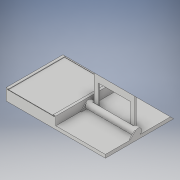
# Autodesk Inventor part: laptop
Saved by Autodesk Inventor 2019.3 (Build 233278000, 278)
## iProperties
Created: 2019-07-12
Part Number: laptop
Material: Generic
Document SubType Name: Modeling
Designer: Frienddo
Density: 1 g/cm^3
Appearance: Default
Author: Frienddo
Autodesk Inventor part; units mm, degrees
ref_plane "YZ Plane" through (0, 0, 0) normal (1, 0, 0) x (0, 1, 0)
sketch "Sketch1" plane through (0, 0, 0) normal (0, 1, 0) x (-1, 0, 0)
  line L0 (-172.25, 111.75) -> (172.25, 111.75)
  line L1 (172.25, 111.75) -> (172.25, -111.75)
  line L2 (172.25, -111.75) -> (-172.25, -111.75)
  line L3 (-172.25, -111.75) -> (-172.25, 111.75)
  line L4 (-172.25, 111.75) -> (172.25, -111.75) construction
  line L5 (172.25, 111.75) -> (-172.25, -111.75) construction
  line L6 (53.000669, 92.142184) -> (35.000669, 92.142184)
  line L7 (35.000669, 92.142184) -> (35.000669, -3.857816)
  line L8 (35.000669, -3.857816) -> (53.000669, -3.857816)
  line L9 (53.000669, -3.857816) -> (53.000669, 92.142184)
  circle A0 centre (38.000669, 83.642184) radius 1.5
  circle A1 centre (38.000669, 44.642184) radius 1.5
  circle A2 centre (38.000669, 7.642184) radius 1.5
  line L10 (146.634879, 91) -> (109.634879, 91)
  line L11 (109.634879, 91) -> (109.634879, -91)
  line L12 (109.634879, -91) -> (146.634879, -91)
  line L13 (146.634879, -91) -> (146.634879, 91)
  circle A3 centre (128.134879, 88.5) radius 1.5
  circle A4 centre (128.134879, -46.5) radius 1.5
  line L14 (89.662991, 91.78307) -> (71.662991, 91.78307)
  line L15 (71.662991, 91.78307) -> (71.662991, 57.78307)
  line L16 (71.662991, 57.78307) -> (89.662991, 57.78307)
  line L17 (89.662991, 57.78307) -> (89.662991, 91.78307)
  circle A5 centre (75.162991, 61.28307) radius 1.5
  circle A6 centre (86.162991, 86.28307) radius 1.5
  line L18 (96.694957, 29.854955) -> (71.694957, 29.854955)
  line L19 (71.694957, 29.854955) -> (71.694957, -90.145045)
  line L20 (71.694957, -90.145045) -> (96.694957, -90.145045)
  line L21 (96.694957, -90.145045) -> (96.694957, 29.854955)
  circle A7 centre (93.194957, -86.645045) radius 1.5
  circle A8 centre (93.194957, 26.354955) radius 1.5
  line L22 (-246.75, 0) -> (246.75, 0)
  line L23 (176.25, -115.75) -> (176.25, 115.75)
  line L24 (176.25, 115.75) -> (-176.25, 115.75)
  line L25 (-176.25, 115.75) -> (-176.25, -115.75)
  line L26 (-176.25, -115.75) -> (176.25, -115.75)
  line L27 (56.000669, 95.142184) -> (32.000669, 95.142184)
  line L28 (32.000669, 95.142184) -> (32.000669, -6.857816)
  line L29 (32.000669, -6.857816) -> (56.000669, -6.857816)
  line L30 (56.000669, -6.857816) -> (56.000669, 95.142184)
  line L31 (92.662991, 94.78307) -> (68.662991, 94.78307)
  line L32 (68.662991, 94.78307) -> (68.662991, 54.78307)
  line L33 (68.662991, 54.78307) -> (92.662991, 54.78307)
  line L34 (92.662991, 54.78307) -> (92.662991, 94.78307)
  line L35 (149.634879, 94) -> (106.634879, 94)
  line L36 (106.634879, 94) -> (106.634879, -94)
  line L37 (106.634879, -94) -> (149.634879, -94)
  line L38 (149.634879, -94) -> (149.634879, 94)
  line L39 (68.694957, 32.854955) -> (99.694957, 32.854955)
  line L40 (99.694957, 32.854955) -> (99.694957, -93.145045)
  line L41 (99.694957, -93.145045) -> (68.694957, -93.145045)
  line L42 (68.694957, -93.145045) -> (68.694957, 32.854955)
  line L43 (56.000669, -93.145045) -> (36.000669, -93.145045)
  line L44 (36.000669, -93.145045) -> (36.000669, -60.178685)
  line L45 (36.000669, -60.178685) -> (56.000669, -60.178685)
  line L46 (56.000669, -60.178685) -> (56.000669, -93.145045)
  point P0 (0, 0)
  dimension "d0" = 344.5
  dimension "d1" = 223.5
  dimension "d4" = 18
  dimension "d5" = 96
  dimension "d6" = 3
  dimension "d7" = 3
  dimension "d8" = 8.5
  dimension "d9" = 3
  dimension "d10" = 47.5
  dimension "d11" = 3
  dimension "d12" = 11.5
  dimension "d13" = 3
  dimension "d14" = 3
  dimension "d15" = 37
  dimension "d16" = 182
  dimension "d17" = 3
  dimension "d18" = 2.5
  dimension "d19" = 18.5
  dimension "d20" = 3
  dimension "d21" = 44.5
  dimension "d23" = 34
  dimension "d24" = 18
  dimension "d25" = 3
  dimension "d26" = 3.5
  dimension "d27" = 3.5
  dimension "d28" = 3
  dimension "d29" = 3.5
  dimension "d30" = 5.5
  dimension "d31" = 25
  dimension "d32" = 120
  dimension "d33" = 3
  dimension "d34" = 3.5
  dimension "d36" = 3
  dimension "d38" = 3.5
  dimension "d39" = 4
  dimension "d42" = 3
  dimension "d43" = 3
  dimension "d44" = 3
  dimension "d67" = 3
  dimension "d68" = 3.5
  dimension "d69" = 3.5
  dimension "d70" = 18.5
  dimension "d94" = 20
  constraints: 92 end point, 22 parallel, 11 perpendicular, 9 centre point, 6 horizontal, 2 midpoint, 16 other
  measures "d0" distance of L1.end L2.end
  measures "d1" distance of L2.end L0.start
  measures "d4" distance of L8.end L7.end
  measures "d5" distance of L6.end L7.end
  measures "d6" diameter of A0
  measures "d7" distance from line of L7 A0.centre
  measures "d8" distance from line of L6 A0.centre
  measures "d9" diameter of A1
  measures "d10" distance from line of L6 A1.centre
  measures "d11" diameter of A2
  measures "d12" distance from line of L8 A2.centre
  measures "d13" distance from line of L7 A2.centre
  measures "d14" distance from line of L7 A1.centre
  measures "d15" distance of L12.end L11.end
  measures "d16" distance of L12.end L10.start
  measures "d17" diameter of A3
  measures "d18" distance from line of L10 A3.centre
  measures "d19" distance from line of L13 A3.centre
  measures "d20" diameter of A4
  measures "d21" distance from line of L12 A4.centre
  measures "d23" distance of L16.end L14.start
  measures "d24" distance of L15.end L16.end
  measures "d25" diameter of A5
  measures "d26" distance from line of L15 A5.centre
  measures "d27" distance from line of L16 A5.centre
  measures "d28" diameter of A6
  measures "d29" distance from line of L17 A6.centre
  measures "d30" distance from line of L14 A6.centre
  measures "d31" distance of L20.end L19.end
  measures "d32" distance of L18.end L19.end
  measures "d33" diameter of A7
  measures "d34" distance from line of L20 A7.centre
  measures "d36" diameter of A8
  measures "d38" distance from line of L18 A8.centre
  measures "d39" distance between parallel lines of L1 L23
  measures "d42" distance between parallel lines of L9 L30
  measures "d43" distance between parallel lines of L17 L34
  measures "d44" distance between parallel lines of L13 L38
  measures "d67" distance between parallel lines of L18 L39
  measures "d68" distance from line of L21 A7.centre
  measures "d69" distance from line of L21 A8.centre
  measures "d70" distance from line of L13 A4.centre
  measures "d94" distance of L44.end L45.end
sketch "Sketch1 outline for Extrusion2" plane through (0, 0, 0) normal (0, 1, 0) x (-1, 0, 0)
  line L0 (-176.25, -115.75) -> (176.25, -115.75)
  line L1 (-176.25, 115.75) -> (-176.25, -115.75)
  line L2 (176.25, 115.75) -> (-176.25, 115.75)
  line L3 (176.25, -115.75) -> (176.25, 115.75)
extrude "Extrusion2" add sketch "Sketch1 outline for Extrusion2" against normal blind 2
sketch "Sketch1 outline for Extrusion3" plane through (0, 0, 0) normal (0, 1, 0) x (-1, 0, 0)
  line L0 (92.662991, 54.78307) -> (92.662991, 94.78307)
  line L1 (68.662991, 54.78307) -> (92.662991, 54.78307)
  line L2 (92.662991, 94.78307) -> (68.662991, 94.78307)
  line L3 (68.662991, 94.78307) -> (68.662991, 54.78307)
  circle A0 centre (75.162991, 61.28307) radius 1.5
  circle A1 centre (86.162991, 86.28307) radius 1.5
  line L4 (56.000669, -6.857816) -> (56.000669, 95.142184)
  line L5 (32.000669, -6.857816) -> (56.000669, -6.857816)
  line L6 (56.000669, 95.142184) -> (32.000669, 95.142184)
  line L7 (32.000669, 95.142184) -> (32.000669, -6.857816)
  circle A2 centre (38.000669, 44.642184) radius 1.5
  circle A3 centre (38.000669, 7.642184) radius 1.5
  circle A4 centre (38.000669, 83.642184) radius 1.5
  line L8 (68.694957, 32.854955) -> (99.694957, 32.854955)
  line L9 (68.694957, -93.145045) -> (68.694957, 32.854955)
  line L10 (99.694957, 32.854955) -> (99.694957, -93.145045)
  line L11 (99.694957, -93.145045) -> (68.694957, -93.145045)
  circle A5 centre (93.194957, -86.645045) radius 1.5
  line L12 (149.634879, -94) -> (149.634879, 94)
  line L13 (106.634879, -94) -> (149.634879, -94)
  line L14 (149.634879, 94) -> (106.634879, 94)
  line L15 (106.634879, 94) -> (106.634879, -94)
  circle A6 centre (128.134879, -46.5) radius 1.5
  circle A7 centre (128.134879, 88.5) radius 1.5
extrude "Extrusion3" add sketch "Sketch1 outline for Extrusion3" along normal blind 5
sketch "Sketch1 outline for Extrusion4" plane through (0, 0, 0) normal (0, 1, 0) x (-1, 0, 0)
  circle A0 centre (93.194957, -86.645045) radius 1.5
  circle A1 centre (93.194957, 26.354955) radius 1.5
extrude "Extrusion4" cut sketch "Sketch1 outline for Extrusion4" along normal blind 6
sketch "Sketch3" plane through (-32.000669, 0, -6.857816) normal (1, 0, 0) x (0, 0, -1)
  line L0 (-92, 0) -> (-92, 5) projected
  line L1 (-89, 0) -> (-89, 5) projected
  line L2 (-53, 0) -> (-53, 5) projected
  line L3 (-50, 0) -> (-50, 5) projected
  line L4 (-16, 0) -> (-16, 5) projected
  line L5 (-13, 0) -> (-13, 5) projected
  line L6 (-92, 0) -> (-89, 0)
  line L7 (-89, 0) -> (-89, 3)
  line L8 (-89, 3) -> (-92, 3)
  line L9 (-92, 3) -> (-92, 0)
  line L10 (-53, 3) -> (-50, 3)
  line L11 (-50, 3) -> (-50, 0)
  line L12 (-50, 0) -> (-53, 0)
  line L13 (-53, 0) -> (-53, 3)
  line L14 (-16, 3) -> (-13, 3)
  line L15 (-13, 3) -> (-13, 0)
  line L16 (-13, 0) -> (-16, 0)
  line L17 (-16, 0) -> (-16, 3)
  point P0 (-6.857816, 0)
  dimension "d49" = 3
  constraints: 24 end point, 6 parallel, 4 point on line, 3 horizontal, 3 perpendicular
  measures "d49" distance between parallel lines of L6 L8
sketch "Sketch3 outline for Extrusion5" plane through (-32.000669, 0, -6.857816) normal (1, 0, 0) x (0, 0, -1)
  line L0 (-92, 3) -> (-92, 0)
  line L1 (-89, 3) -> (-92, 3)
  line L2 (-89, 0) -> (-89, 3)
  line L3 (-92, 0) -> (-89, 0)
  line L4 (-53, 0) -> (-50, 0)
  line L5 (-53, 3) -> (-53, 0)
  line L6 (-50, 3) -> (-53, 3)
  line L7 (-50, 0) -> (-50, 3)
  line L8 (-16, 0) -> (-13, 0)
  line L9 (-16, 3) -> (-16, 0)
  line L10 (-13, 3) -> (-16, 3)
  line L11 (-13, 0) -> (-13, 3)
extrude "Extrusion5" cut sketch "Sketch3 outline for Extrusion5" against normal blind 6
sketch "Sketch4" plane through (-99.694957, 0, -90.145045) normal (1, 0, 0) x (0, 0, -1)
  line L0 (-115, 0) -> (-115, 5) projected
  line L1 (-118, 0) -> (-118, 5) projected
  line L2 (-5, 0) -> (-5, 5) projected
  line L3 (-5, 5) -> (-2, 5) projected
  line L4 (-2, 0) -> (-2, 5) projected
  line L5 (-118, 0) -> (-115, 0)
  line L6 (-115, 0) -> (-115, 3)
  line L7 (-115, 3) -> (-118, 3)
  line L8 (-118, 3) -> (-118, 0)
  line L9 (-5, 0) -> (-2, 0)
  line L10 (-2, 0) -> (-2, 3)
  line L11 (-2, 3) -> (-5, 3)
  line L12 (-5, 3) -> (-5, 0)
  point P0 (-90.145045, 0)
  dimension "d52" = 3
  constraints: 16 end point, 4 parallel, 2 horizontal, 2 perpendicular, 2 point on line
  measures "d52" distance between parallel lines of L5 L7
sketch "Sketch4 outline for Extrusion6" plane through (-99.694957, 0, -90.145045) normal (1, 0, 0) x (0, 0, -1)
  line L0 (-118, 3) -> (-118, 0)
  line L1 (-115, 3) -> (-118, 3)
  line L2 (-115, 0) -> (-115, 3)
  line L3 (-118, 0) -> (-115, 0)
  line L4 (-5, 3) -> (-5, 0)
  line L5 (-2, 3) -> (-5, 3)
  line L6 (-2, 0) -> (-2, 3)
  line L7 (-5, 0) -> (-2, 0)
extrude "Extrusion6" cut sketch "Sketch4 outline for Extrusion6" along normal blind 6.5
sketch "Sketch5" plane through (-68.662991, 0, 54.78307) normal (1, 0, 0) x (0, 0, -1)
  line L0 (-5, 0) -> (-5, 5) projected
  line L1 (-8, 0) -> (-8, 5) projected
  line L2 (-8, 0) -> (-5, 0)
  line L3 (-5, 0) -> (-5, 3)
  line L4 (-5, 3) -> (-8, 3)
  line L5 (-8, 3) -> (-8, 0)
  point P0 (54.78307, 0)
  dimension "d55" = 3
  constraints: 8 end point, 2 parallel, 1 horizontal, 1 perpendicular, 1 point on line
  measures "d55" distance between parallel lines of L2 L4
sketch "Sketch5 outline for Extrusion7" plane through (-68.662991, 0, 54.78307) normal (1, 0, 0) x (0, 0, -1)
  line L0 (-8, 3) -> (-8, 0)
  line L1 (-5, 3) -> (-8, 3)
  line L2 (-5, 0) -> (-5, 3)
  line L3 (-8, 0) -> (-5, 0)
extrude "Extrusion7" cut sketch "Sketch5 outline for Extrusion7" against normal blind 6.5
sketch "Sketch6" plane through (-92.662991, 0, 94.78307) normal (-1, 0, 0) x (0, 0, 1)
  line L0 (-7, 0) -> (-7, 5) projected
  line L1 (-10, 0) -> (-10, 5) projected
  line L2 (-7, 0) -> (-10, 0)
  line L3 (-10, 0) -> (-10, 3)
  line L4 (-10, 3) -> (-7, 3)
  line L5 (-7, 3) -> (-7, 0)
  point P0 (-94.78307, 0)
  dimension "d58" = 3
  constraints: 8 end point, 2 parallel, 1 horizontal, 1 perpendicular, 1 point on line
  measures "d58" distance of L4.end L0.start
sketch "Sketch6 outline for Extrusion8" plane through (-92.662991, 0, 94.78307) normal (-1, 0, 0) x (0, 0, 1)
  line L0 (-7, 0) -> (-10, 0)
  line L1 (-10, 0) -> (-10, 3)
  line L2 (-10, 3) -> (-7, 3)
  line L3 (-7, 3) -> (-7, 0)
extrude "Extrusion8" cut sketch "Sketch6 outline for Extrusion8" against normal blind 6.5
sketch "Sketch7" plane through (-149.634879, 0, 94) normal (0, 0, 1) x (1, 0, 0)
  line L0 (20, 0) -> (20, 5) projected
  line L1 (23, 0) -> (23, 5) projected
  line L2 (20, 3) -> (23, 3)
  line L3 (23, 3) -> (23, 0)
  line L4 (23, 0) -> (20, 0)
  line L5 (20, 0) -> (20, 3)
  point P0 (149.634879, 0)
  dimension "d61" = 3
  constraints: 8 end point, 2 parallel, 1 horizontal, 1 perpendicular, 1 point on line
  measures "d61" distance between parallel lines of L4 L2
sketch "Sketch7 outline for Extrusion9" plane through (-149.634879, 0, 94) normal (0, 0, 1) x (1, 0, 0)
  line L0 (20, 0) -> (23, 0)
  line L1 (20, 3) -> (20, 0)
  line L2 (23, 3) -> (20, 3)
  line L3 (23, 0) -> (23, 3)
extrude "Extrusion9" cut sketch "Sketch7 outline for Extrusion9" against normal blind 5.5
sketch "Sketch8" plane through (-106.634879, 0, -94) normal (1, 0, 0) x (0, 0, -1)
  line L0 (-49, 0) -> (-49, 5) projected
  line L1 (-46, 0) -> (-46, 5) projected
  line L2 (-49, 0) -> (-46, 0)
  line L3 (-46, 0) -> (-46, 3)
  line L4 (-46, 3) -> (-49, 3)
  line L5 (-49, 3) -> (-49, 0)
  point P0 (-94, 0)
  dimension "d64" = 3
  constraints: 8 end point, 2 parallel, 1 horizontal, 1 perpendicular, 1 point on line
  measures "d64" distance between parallel lines of L2 L4
sketch "Sketch8 outline for Extrusion10" plane through (-106.634879, 0, -94) normal (1, 0, 0) x (0, 0, -1)
  line L0 (-49, 3) -> (-49, 0)
  line L1 (-46, 3) -> (-49, 3)
  line L2 (-46, 0) -> (-46, 3)
  line L3 (-49, 0) -> (-46, 0)
extrude "Extrusion10" cut sketch "Sketch8 outline for Extrusion10" against normal up to next
sketch "Sketch9" plane through (-176.25, 0, -115.75) normal (-1, 0, 0) x (0, 0, 1)
  line L0 (231.5, 0) -> (231.5, -2) projected
  line L1 (231.5, 0) -> (231.5, 30)
  line L2 (0, 0) -> (231.5, 0) projected
  line L3 (0, 0) -> (30, 30)
  line L4 (30, 30) -> (231.5, 30)
  line L5 (0, 0) -> (231.5, 0)
  line L6 (21.75, 5) -> (209.75, 5) projected
  line L7 (189.25, 20) -> (200.25, 20)
  line L8 (200.25, 20) -> (200.25, 3)
  line L9 (200.25, 3) -> (189.25, 3)
  line L10 (189.25, 3) -> (189.25, 20)
  line L11 (189.25, 20) -> (200.25, 3) construction
  line L12 (200.25, 20) -> (189.25, 3) construction
  line L13 (137.75, 17) -> (157.75, 17)
  line L14 (157.75, 17) -> (157.75, 3)
  line L15 (157.75, 3) -> (137.75, 3)
  line L16 (137.75, 3) -> (137.75, 17)
  line L17 (137.75, 17) -> (157.75, 3) construction
  line L18 (157.75, 17) -> (137.75, 3) construction
  point P0 (115.75, 0)
  point P1 (194.75, 11.5)
  point P2 (147.75, 10)
  dimension "d71" = 30
  dimension "d72" = 45
  dimension "d100" = 15
  dimension "d101" = 62
  dimension "d102" = 17
  dimension "d103" = 14
  dimension "d104" = 20
  dimension "d105" = 2
  dimension "d106" = 2
  dimension "d107" = 11
  constraints: 32 end point, 4 horizontal, 4 midpoint, 4 parallel, 2 perpendicular, 1 vertical
  measures "d71" distance of L0.start L1.end
  measures "d72" angle of L2 L3
  measures "d100" horizontal distance of L6.end point (194.75, 11.5)
  measures "d101" horizontal distance of L6.end point (147.75, 10)
  measures "d102" distance of L7.end L8.end
  measures "d103" distance of L13.end L14.end
  measures "d104" distance of L13.start L13.end
  measures "d105" distance between parallel lines of L15 L6
  measures "d106" distance between parallel lines of L9 L6
  measures "d107" distance of L7.start L7.end
sketch "Sketch9 outline for Extrusion11" plane through (-176.25, 0, -115.75) normal (-1, 0, 0) x (0, 0, 1)
  line L0 (0, 0) -> (231.5, 0)
  line L1 (30, 30) -> (0, 0)
  line L2 (231.5, 30) -> (30, 30)
  line L3 (231.5, 0) -> (231.5, 30)
extrude "Extrusion11" add sketch "Sketch9 outline for Extrusion11" against normal blind 4
sketch "Sketch9 outline for Extrusion12" plane through (-176.25, 0, -115.75) normal (-1, 0, 0) x (0, 0, 1)
  line L0 (0, 0) -> (231.5, 0)
  line L1 (30, 30) -> (0, 0)
  line L2 (231.5, 30) -> (30, 30)
  line L3 (231.5, 0) -> (231.5, 30)
extrude "Extrusion12" add sketch "Sketch9 outline for Extrusion12" along normal blind 4 from surface at -176.25
sketch "Sketch10" plane through (0, 0, -115.75) normal (0, 0.7071068, -0.7071068) x (-1, 0, 0)
  line L0 (0, 0) -> (0, 163.69522)
  line L1 (176.25, 42.426407) -> (176.25, 0)
  line L2 (0, 0) -> (176.25, 0)
  line L3 (176.25, 0) -> (176.25, 42.426407)
  line L4 (176.25, 42.426407) -> (0, 42.426407)
  line L5 (0, 42.426407) -> (0, 0)
  point P0 (0, 81.84761)
  constraints: 8 end point, 2 parallel, 1 horizontal, 1 perpendicular
sketch "Sketch10 outline for Extrusion13" plane through (0, 0, -115.75) normal (0, 0.7071068, -0.7071068) x (-1, 0, 0)
  line L0 (0, 42.426407) -> (0, 0)
  line L1 (176.25, 42.426407) -> (0, 42.426407)
  line L2 (176.25, 0) -> (176.25, 42.426407)
  line L3 (0, 0) -> (176.25, 0)
extrude "Extrusion13" add sketch "Sketch10 outline for Extrusion13" against normal blind 4
sketch "Sketch11" plane through (-176.25, -2, 115.75) normal (0, 0, 1) x (1, 0, 0)
  line L0 (172.25, 32) -> (167.25, 32)
  line L1 (167.25, 32) -> (167.25, 30)
  line L2 (167.25, 30) -> (171.25, 30)
  line L3 (171.25, 30) -> (171.25, 27.5)
  line L4 (171.25, 27.5) -> (167.25, 27.5)
  line L5 (167.25, 27.5) -> (167.25, 25.5)
  line L6 (167.25, 25.5) -> (172.25, 25.5)
  line L7 (172.25, 2) -> (172.25, 32)
  line L8 (176.25, 32) -> (172.25, 32)
  line L9 (172.25, 32) -> (172.25, 25.5)
  line L10 (4, 32) -> (4, 2)
  line L11 (172.25, 17) -> (4, 17) construction
  line L12 (88.125, 17) -> (88.125, 10.810399) construction
  line L13 (4, 32) -> (9, 32)
  line L14 (9, 32) -> (9, 30)
  line L15 (9, 30) -> (5, 30)
  line L16 (5, 30) -> (5, 27.5)
  line L17 (5, 27.5) -> (9, 27.5)
  line L18 (9, 27.5) -> (9, 25.5)
  line L19 (9, 25.5) -> (4, 25.5)
  line L20 (4, 2) -> (4, 32)
  line L21 (0, 32) -> (4, 32)
  line L22 (4, 32) -> (4, 25.5)
  line L23 (4, 17) -> (172.25, 17) construction
  point P0 (176.25, 2)
  dimension "d79" = 2
  dimension "d80" = 2
  dimension "d81" = 2.5
  dimension "d82" = 4
  dimension "d83" = 1
  constraints: 42 end point, 10 symmetric about line, 6 perpendicular, 6 point on line, 3 midpoint, 1 horizontal, 1 vertical
  measures "d79" distance between parallel lines of L0 L2
  measures "d80" distance between parallel lines of L4 L6
  measures "d81" distance between parallel lines of L2 L4
  measures "d82" distance between parallel lines of L5 L3
  measures "d83" distance between parallel lines of L7 L3
sketch "Sketch11 outline for Extrusion14" plane through (-176.25, -2, 115.75) normal (0, 0, 1) x (1, 0, 0)
  line L0 (172.25, 25.5) -> (172.25, 32)
  line L1 (167.25, 25.5) -> (172.25, 25.5)
  line L2 (167.25, 27.5) -> (167.25, 25.5)
  line L3 (171.25, 27.5) -> (167.25, 27.5)
  line L4 (171.25, 30) -> (171.25, 27.5)
  line L5 (167.25, 30) -> (171.25, 30)
  line L6 (167.25, 32) -> (167.25, 30)
  line L7 (172.25, 32) -> (167.25, 32)
  line L8 (4, 32) -> (9, 32)
  line L9 (9, 32) -> (9, 30)
  line L10 (9, 30) -> (5, 30)
  line L11 (5, 30) -> (5, 27.5)
  line L12 (5, 27.5) -> (9, 27.5)
  line L13 (9, 27.5) -> (9, 25.5)
  line L14 (9, 25.5) -> (4, 25.5)
  line L15 (4, 25.5) -> (4, 32)
extrude "Extrusion14" add sketch "Sketch11 outline for Extrusion14" against normal up to next
sketch "Sketch12" plane through (-176.25, -2, 115.75) normal (0, 0, 1) x (1, 0, 0)
  line L0 (172.25, 27.5) -> (4, 27.5)
  line L1 (4, 27.5) -> (4, 2)
  line L2 (4, 2) -> (172.25, 2)
  line L3 (172.25, 2) -> (172.25, 27.5)
  line L4 (172.25, 2) -> (172.25, 25.5) projected
  constraints: 8 end point, 2 parallel, 1 collinear, 1 horizontal, 1 perpendicular
sketch "Sketch12 outline for Extrusion15" plane through (-176.25, -2, 115.75) normal (0, 0, 1) x (1, 0, 0)
  line L0 (4, 2) -> (4, 27.5)
  line L1 (4, 27.5) -> (172.25, 27.5)
  line L2 (172.25, 27.5) -> (172.25, 2)
  line L3 (172.25, 2) -> (4, 2)
extrude "Extrusion15" add sketch "Sketch12 outline for Extrusion15" against normal blind 4
sketch "Sketch13" plane through (-5, 25.5, -84.593146) normal (-1, 0, 0) x (0, 0, 1)
  line L0 (200.343146, 2.5) -> (0.843146, 2.5)
  line L1 (200.343146, 2.5) -> (200.343146, 0)
  line L2 (0.843146, 2.5) -> (200.343146, 2.5)
  line L3 (200.343146, 2.5) -> (200.343146, 0)
  line L4 (200.343146, 0) -> (0.843146, 0)
  line L5 (0.843146, 0) -> (0.843146, 2.5)
  point P0 (84.593146, -25.5)
  constraints: 8 end point, 2 parallel, 1 horizontal, 1 perpendicular
sketch "Sketch13 outline for Extrusion16" plane through (-5, 25.5, -84.593146) normal (-1, 0, 0) x (0, 0, 1)
  line L0 (200.343146, 2.5) -> (0.843146, 2.5)
  line L1 (200.343146, 0) -> (200.343146, 2.5)
  line L2 (0.843146, 0) -> (200.343146, 0)
  line L3 (0.843146, 2.5) -> (0.843146, 0)
extrude "Extrusion16" cut sketch "Sketch13 outline for Extrusion16" along normal up to surface (166.25 mm away)
sketch "Sketch14" plane through (-176.25, -2, 115.75) normal (-1, 0, 0) x (0, 0, 1)
  line L0 (-229.5, 0) -> (-228.671573, -0.828427)
  line L1 (-227.843146, 0) -> (-229.5, 0)
  line L2 (-229.5, 0) -> (-227.843146, 0)
  line L3 (-228.671573, -0.828427) -> (-227.843146, 0)
  line L4 (-227.843146, 0) -> (-228.671573, -0.828427)
  line L5 (-228.671573, -0.828427) -> (-229.5, 0)
  point P0 (-115.75, 2)
  constraints: 6 end point, 1 collinear, 1 horizontal, 1 perpendicular
sketch "Sketch14 outline for Extrusion17" plane through (-176.25, -2, 115.75) normal (-1, 0, 0) x (0, 0, 1)
  line L0 (-227.843146, 0) -> (-229.5, 0)
  line L1 (-228.671573, -0.828427) -> (-227.843146, 0)
  line L2 (-229.5, 0) -> (-228.671573, -0.828427)
extrude "Extrusion17" cut sketch "Sketch14 outline for Extrusion17" against normal through all
sketch "Sketch1 outline for Extrusion18" plane through (0, 0, 0) normal (0, 1, 0) x (-1, 0, 0)
  line L0 (-176.25, -115.75) -> (176.25, -115.75)
  line L1 (-176.25, 115.75) -> (-176.25, -115.75)
  line L2 (176.25, -115.75) -> (176.25, 115.75)
  line L3 (176.25, 115.75) -> (-176.25, 115.75)
  line L4 (-172.25, -111.75) -> (-172.25, 111.75)
  line L5 (172.25, -111.75) -> (-172.25, -111.75)
  line L6 (172.25, 111.75) -> (172.25, -111.75)
  line L7 (-172.25, 111.75) -> (172.25, 111.75)
extrude "Extrusion18" add sketch "Sketch1 outline for Extrusion18" against normal blind 8.6
sketch "Sketch1 outline for Extrusion19" plane through (0, 0, 0) normal (0, 1, 0) x (-1, 0, 0)
  line L0 (56.000669, -93.145045) -> (36.000669, -93.145045)
  line L1 (36.000669, -93.145045) -> (36.000669, -60.178685)
  line L2 (36.000669, -60.178685) -> (56.000669, -60.178685)
  line L3 (56.000669, -60.178685) -> (56.000669, -93.145045)
extrude "Extrusion19" cut sketch "Sketch1 outline for Extrusion19" against normal through all
sketch "Sketch15" plane through (0, -8.6, 0) normal (0, -1, 0) x (1, 0, 0)
  line L0 (-176.25, 115.75) -> (-167.25, 115.75) projected
  line L1 (176.25, 115.75) -> (176.25, -115.75) projected
  line L2 (-176.25, 115.75) -> (176.25, 115.75)
  line L3 (176.25, 115.75) -> (176.25, -115.75)
  line L4 (176.25, -115.75) -> (-176.25, -115.75)
  line L5 (-176.25, -115.75) -> (-176.25, 115.75)
  line L6 (169.25, 108.75) -> (-169.25, 108.75)
  line L7 (-169.25, 108.75) -> (-169.25, -108.75)
  line L8 (-169.25, -108.75) -> (169.25, -108.75)
  line L9 (169.25, -108.75) -> (169.25, 108.75)
  point P0 (0, 0)
  dimension "d97" = 7
  constraints: 16 end point, 4 parallel, 2 perpendicular, 1 horizontal, 3 other
  measures "d97" distance between parallel lines of L2 L6
sketch "Sketch15 outline for Extrusion20" plane through (0, -8.6, 0) normal (0, -1, 0) x (1, 0, 0)
  line L0 (-176.25, 115.75) -> (176.25, 115.75)
  line L1 (-176.25, -115.75) -> (-176.25, 115.75)
  line L2 (176.25, 115.75) -> (176.25, -115.75)
  line L3 (176.25, -115.75) -> (-176.25, -115.75)
  line L4 (169.25, -108.75) -> (169.25, 108.75)
  line L5 (169.25, 108.75) -> (-169.25, 108.75)
  line L6 (-169.25, 108.75) -> (-169.25, -108.75)
  line L7 (-169.25, -108.75) -> (169.25, -108.75)
extrude "Extrusion20" add sketch "Sketch15 outline for Extrusion20" along normal blind 3
sketch "Sketch9 outline for Extrusion21" plane through (-176.25, 0, -115.75) normal (-1, 0, 0) x (0, 0, 1)
  line L0 (189.25, 20) -> (200.25, 20)
  line L1 (200.25, 20) -> (200.25, 3)
  line L2 (200.25, 3) -> (189.25, 3)
  line L3 (189.25, 3) -> (189.25, 20)
  line L4 (137.75, 17) -> (157.75, 17)
  line L5 (157.75, 17) -> (157.75, 3)
  line L6 (157.75, 3) -> (137.75, 3)
  line L7 (137.75, 3) -> (137.75, 17)
extrude "Extrusion21" cut sketch "Sketch9 outline for Extrusion21" against normal up to surface (4 mm away)
sketch "Sketch17" plane through (176.25, 0, 115.75) normal (1, 0, 0) x (0, 0, -1)
  line L0 (231.5, 0) -> (231.5, -11.6) projected
  line L1 (231.5, -11.6) -> (231.5, 0)
  line L2 (231.5, 0) -> (243.1, -11.6)
  line L3 (243.1, -11.6) -> (231.5, -11.6)
  point P0 (115.75, 0)
  dimension "d111" = 45
  constraints: 6 end point, 1 collinear, 1 perpendicular
  measures "d111" angle of L3 L2
sketch "Sketch17 outline for Extrusion22" plane through (176.25, 0, 115.75) normal (1, 0, 0) x (0, 0, -1)
  line L0 (243.1, -11.6) -> (231.5, 0)
  line L1 (231.5, -11.6) -> (243.1, -11.6)
  line L2 (231.5, 0) -> (231.5, -11.6)
extrude "Extrusion22" add sketch "Sketch17 outline for Extrusion22" against normal up to surface (352.5 mm away)
sketch "Sketch16" plane through (176.25, 0, 115.75) normal (1, 0, 0) x (0, 0, -1)
  arc A0 (115.75, 0) -> (115.75, 20) centre (115.75, 10) ccw
  line L0 (0, 0) -> (231.5, 0)
  arc A1 (107.443376, 0) -> (115.75, 23) centre (115.75, 10) ccw
  line L1 (87.365224, 0) -> (106.557612, 19.192388)
  line L2 (115.75, 0) -> (115.75, 35.556642) construction
  arc A2 (106.557612, 19.192388) -> (107.443376, 0) centre (115.75, 10) ccw
  line L3 (87.365224, 0) -> (107.443376, 0)
  line L4 (227.5, -2) -> (4, -2)
  arc A3 (115.75, 20) -> (115.75, 0) centre (115.75, 10) ccw
  arc A4 (115.75, 23) -> (106.557612, 19.192388) centre (115.75, 10) ccw
  line L5 (115.25, 19.987492) -> (115.25, 22.990381)
  point P0 (124.942388, 19.192388)
  point P1 (139.134776, 0)
  dimension "d110" = 20
  dimension "d114" = 3
  dimension "d115" = 45
  dimension "d131" = 0.5
  constraints: 14 point on circle, 8 end point, 6 point on line, 5 centre point, 3 tangent, 2 vertical, 1 midpoint, 1 parallel
  measures "d110" diameter of A0
  measures "d114" radial gap between concentric circles of A0 A1
  measures "d115" angle of L2 L1
  measures "d131" distance between parallel lines of L2 L5
sketch "Sketch16 outline for Extrusion25" plane through (176.25, 0, 115.75) normal (1, 0, 0) x (0, 0, -1)
  line L0 (87.365224, 0) -> (106.557612, 19.192388)
  arc A0 (106.557612, 19.192388) -> (115.75, 23) centre (115.75, 10) cw
  arc A1 (115.75, 23) -> (107.443376, 0) centre (115.75, 10) cw
  line L1 (107.443376, 0) -> (87.365224, 0)
extrude "Extrusion25" add sketch "Sketch16 outline for Extrusion25" against normal blind 3
sketch "Sketch16 outline for Extrusion26" plane through (176.25, 0, 115.75) normal (1, 0, 0) x (0, 0, -1)
  circle A0 centre (115.75, 10) radius 13
  circle A1 centre (115.75, 10) radius 10
extrude "Extrusion26" add sketch "Sketch16 outline for Extrusion26" against normal blind 15
ref_plane "Work Plane1" through (88.125, 0, 115.75) normal (1, 0, 0) x (0, 0, -1)
mirror "Mirror1" about plane through (88.125, 0, 115.75) normal (1, 0, 0) of "Extrusion26", "Extrusion25"
sketch "Sketch16 outline for Extrusion27" plane through (176.25, 0, 115.75) normal (1, 0, 0) x (0, 0, -1)
  line L0 (107.443376, 0) -> (115.75, 0)
  arc A0 (106.557612, 19.192388) -> (107.443376, 0) centre (115.75, 10) ccw
  arc A1 (115.25, 22.990381) -> (106.557612, 19.192388) centre (115.75, 10) ccw
  line L1 (115.25, 19.987492) -> (115.25, 22.990381)
  arc A2 (115.75, 0) -> (115.25, 19.987492) centre (115.75, 10) cw
extrude "Extrusion27" add sketch "Sketch16 outline for Extrusion27" against normal up to surface (161.25 mm away)
ref_plane "Work Plane2" through (15.5, 0, 0) normal (1, 0, 0) x (0, 0, -1)
sketch "Sketch20" plane through (15.5, 0, 0) normal (1, 0, 0) x (0, 0, -1)
  arc A0 (0, 20) -> (0, 0) centre (0, 10) ccw
  arc A1 (0, 0) -> (0, 20) centre (0, 10) ccw
  line L0 (-115.75, 0) -> (115.75, 0)
  line L1 (127.35, -11.6) -> (115.75, 0)
  line L2 (115.75, 0) -> (1.669643, 114.080357)
  circle A2 centre (0, 10) radius 9.6
  line L3 (5.024587, 18.180069) -> (5.024587, 110.725413)
  line L4 (9.6, 10) -> (9.6, 106.15)
  dimension "d132" = 0.4
  dimension "d133" = 45
  constraints: 6 end point, 2 point on circle, 2 point on line, 1 centre point, 1 coincident, 1 collinear, 1 parallel
  measures "d132" radial gap between concentric circles of A2 A1
  measures "d133" angle of L3 L2
sketch "Sketch20 outline for Extrusion29" plane through (15.5, 0, 0) normal (1, 0, 0) x (0, 0, -1)
  line L0 (9.6, 106.15) -> (9.6, 10)
  arc A0 (9.6, 10) -> (5.024587, 18.180069) centre (0, 10) cw
  line L1 (5.024587, 18.180069) -> (5.024587, 110.725413)
  line L2 (5.024587, 110.725413) -> (9.6, 106.15)
extrude "Extrusion29" add sketch "Sketch20 outline for Extrusion29" along normal blind 15
sketch "Sketch20 outline for Extrusion30" plane through (15.5, 0, 0) normal (1, 0, 0) x (0, 0, -1)
  arc A0 (9.6, 10) -> (5.024587, 18.180069) centre (0, 10) cw
  arc A1 (5.024587, 18.180069) -> (9.6, 10) centre (0, 10) cw
extrude "Extrusion30" add sketch "Sketch20 outline for Extrusion30" against normal blind 12
sketch "Sketch21" plane through (30.5, 0, 0) normal (1, 0, 0) x (0, 0, -1)
  line L0 (5.024587, 110.725413) -> (5.024587, 18.180069)
  line L1 (5.024587, 110.725413) -> (5.024587, 89.739485)
  line L2 (9.6, 10) -> (9.6, 106.15)
  line L3 (9.6, 106.15) -> (5.024587, 110.725413)
  line L4 (9.6, 106.15) -> (5.024587, 110.725413)
  line L5 (5.024587, 110.725413) -> (9.6, 106.15)
  line L6 (9.6, 86.725413) -> (5.024587, 86.725413)
  point P0 (0, 0)
  point P1 (9.6, 80.164072)
  dimension "d142" = 24
  constraints: 8 end point, 4 point on line, 2 collinear, 1 perpendicular
  measures "d142" distance of L0.start L6.end
sketch "Sketch21 outline for Extrusion31" plane through (30.5, 0, 0) normal (1, 0, 0) x (0, 0, -1)
  line L0 (9.6, 106.15) -> (5.024587, 110.725413)
  line L1 (9.6, 86.725413) -> (9.6, 106.15)
  line L2 (5.024587, 86.725413) -> (9.6, 86.725413)
  line L3 (5.024587, 89.739485) -> (5.024587, 86.725413)
  line L4 (5.024587, 110.725413) -> (5.024587, 89.739485)
extrude "Extrusion31" add sketch "Sketch21 outline for Extrusion31" along normal up to surface (57.625 mm away)
mirror "Mirror2" about plane through (88.125, 0, 115.75) normal (1, 0, 0) of "Extrusion31", "Extrusion30", "Extrusion29"
chamfer "Chamfer1" distance 5 angle 45 3 edges at (-84.195, 0, 32.855) (-80.663, 0, 94.7831) (-44.0007, 0, 95.1422)
sketch "Sketch24" plane through (-106.634879, 0, -94) normal (1, 0, 0) x (0, 0, -1)
  line L0 (-188, 0) -> (-188, 5) projected
  line L1 (-188, 0) -> (-188, 5)
  line L2 (-188, 5) -> (-193, 0)
  line L3 (-193, 0) -> (-188, 0)
  line L4 (-49, 0) -> (-188, 0) projected
  point P0 (-94, 0)
  dimension "d152" = 45
  constraints: 6 end point, 2 collinear, 1 perpendicular
  measures "d152" angle of L3 L2
sketch "Sketch24 outline for Extrusion34" plane through (-106.634879, 0, -94) normal (1, 0, 0) x (0, 0, -1)
  line L0 (-193, 0) -> (-188, 0)
  line L1 (-188, 5) -> (-193, 0)
  line L2 (-188, 0) -> (-188, 5)
extrude "Extrusion34" add sketch "Sketch24 outline for Extrusion34" against normal up to surface (43 mm away)
sketch "Sketch25" plane through (-126.634879, 3, 94) normal (0, 0, -1) x (-1, 0, 0)
  line L0 (3, -3) -> (3, 0) projected
  line L1 (3, 0) -> (0, 0) projected
  line L2 (0, 0) -> (0, -3) projected
  line L3 (3, -3) -> (0, -3) projected
  point P0 (-126.634879, -3)
sketch "Sketch25 outline for Extrusion35" plane through (-126.634879, 3, 94) normal (0, 0, -1) x (-1, 0, 0)
  line L0 (0, -3) -> (3, -3)
  line L1 (0, 0) -> (0, -3)
  line L2 (3, 0) -> (0, 0)
  line L3 (3, -3) -> (3, 0)
extrude "Extrusion35" cut sketch "Sketch25 outline for Extrusion35" against normal up to surface surface through (-106.634879, 0, 99) normal (0, 0.7071068, 0.7071068)
sketch "Sketch26" plane through (15, 10, 0) normal (1, 0, 0) x (0, 0, -1)
  line L0 (-5, -12) -> (5, -12) projected
  arc A0 (-5, -12) -> (5, -12) centre (0, 0) ccw projected
  point P0 (0, -10)
sketch "Sketch26 outline for Extrusion36" plane through (15, 10, 0) normal (1, 0, 0) x (0, 0, -1)
  line L0 (-5, -12) -> (5, -12)
  arc A0 (5, -12) -> (-5, -12) centre (0, 0) cw
extrude "Extrusion36" cut sketch "Sketch26 outline for Extrusion36" against normal up to surface (15 mm away)
sketch "Sketch27" plane through (161.25, 0, 115.75) normal (-1, 0, 0) x (0, 0, 1)
  line L0 (-120.75, -2) -> (-110.75, -2) projected
  arc A0 (-120.75, -2) -> (-110.75, -2) centre (-115.75, 10) ccw projected
  point P0 (-115.75, 0)
sketch "Sketch27 outline for Extrusion37" plane through (161.25, 0, 115.75) normal (-1, 0, 0) x (0, 0, 1)
  arc A0 (-120.75, -2) -> (-110.75, -2) centre (-115.75, 10) ccw
  line L0 (-110.75, -2) -> (-120.75, -2)
extrude "Extrusion37" cut sketch "Sketch27 outline for Extrusion37" against normal up to surface (11 mm away)
ref_plane "Work Plane3" through (-171.25, 26.343146, -83.35) normal (0, 0, 1) x (1, 0, 0)
sketch "Sketch23" plane through (0, 0, 115.75) normal (0, 0, 1) x (1, 0, 0)
  line L0 (-5, 28) -> (-5, 25.5) projected
  line L1 (-167.25, 28) -> (-171.25, 28) projected
  line L2 (-5, 25.5) -> (-171.25, 25.5)
  line L3 (-171.25, 25.5) -> (-171.25, 28)
  line L4 (-171.25, 28) -> (-5, 28)
  line L5 (-5, 28) -> (-5, 25.5)
  line L6 (-170.75, 26) -> (-5.5, 26)
  line L7 (-5.5, 26) -> (-5.5, 27.5)
  line L8 (-5.5, 27.5) -> (-170.75, 27.5)
  line L9 (-170.75, 27.5) -> (-170.75, 26)
  point P0 (0, 0)
  dimension "d146" = 0.5
  constraints: 16 end point, 4 parallel, 2 perpendicular, 1 horizontal, 3 other
  measures "d146" distance between parallel lines of L2 L6
sketch "Sketch23 outline for Extrusion33" plane through (0, 0, 115.75) normal (0, 0, 1) x (1, 0, 0)
  line L0 (-170.75, 27.5) -> (-170.75, 26)
  line L1 (-5.5, 27.5) -> (-170.75, 27.5)
  line L2 (-5.5, 26) -> (-5.5, 27.5)
  line L3 (-170.75, 26) -> (-5.5, 26)
extrude "Extrusion33" add sketch "Sketch23 outline for Extrusion33" against normal up to surface (199.1 mm away)
body "Solid2"
